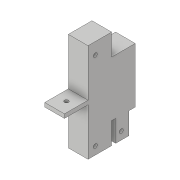
# Autodesk Inventor part: 00_Microlinearmotor
Saved by Autodesk Inventor 2019.4 (Build 234330000, 330)
## iProperties
Created: 2021-09-28
Part Number: 00_Microlinearmotor
Material: Generic
Document SubType Name: Modeling
Designer: diederichbenedict
Density: 1 g/cm^3
Appearance: Default
Author: diederichbenedict
Autodesk Inventor part; units mm, degrees
ref_plane "YZ Plane" through (0, 0, 0) normal (1, 0, 0) x (0, 1, 0)
ref_plane "XZ Plane" through (0, 0, 0) normal (0, 1, 0) x (-1, 0, 0)
ref_plane "XY Plane" through (0, 0, 0) normal (0, 0, 1) x (1, 0, 0)
sketch "Sketch1" plane through (0, 0, 0) normal (1, 0, 0) x (0, 1, 0)
  line L0 (-3.0178, 2.5025) -> (21.9822, 2.5025)
  line L1 (21.9822, 2.5025) -> (21.9822, -3.4975)
  line L2 (21.9822, -3.4975) -> (-3.0178, -3.4975)
  line L3 (-3.0178, -3.4975) -> (-3.0178, 2.5025)
  circle A0 centre (-1.0178, 0.668) radius 0.5
  circle A1 centre (18.9822, 0.668) radius 0.5
  line L4 (16.4822, -3.4975) -> (2.4822, -3.4975)
  line L5 (2.4822, -3.4975) -> (2.4822, -9.4975)
  line L6 (2.4822, -9.4975) -> (16.4822, -9.4975)
  line L7 (9.9822, 2.5025) -> (8.9822, 2.5025)
  line L8 (8.9822, 2.5025) -> (8.9822, 8.5025)
  line L9 (8.9822, 8.5025) -> (9.9822, 8.5025)
  line L10 (9.9822, 8.5025) -> (9.9822, 2.5025)
  line L11 (16.4822, -9.4975) -> (16.4822, -3.4975)
  circle A2 centre (-1.0178, -5.932) radius 0.5
  line L12 (2.4822, -4.5336) -> (-3.0178, -4.5336)
  line L13 (-3.0178, -4.5336) -> (-3.0178, -7.908)
  line L14 (-3.0178, -7.908) -> (2.4822, -7.908)
  line L15 (2.4822, -7.908) -> (2.4822, -4.5336)
  point P0 (0, 0)
  dimension "d0" = 25
  dimension "d1" = 6
  dimension "d2" = 1
  dimension "d3" = 1
  dimension "d4" = 20
  dimension "d5" = 14
  dimension "d6" = 6
  dimension "d8" = 1
  dimension "d9" = 6
  dimension "d10" = 10
  dimension "d13" = 2
  dimension "d18" = 3
  dimension "d19" = 5.5
  dimension "d20" = 1
  dimension "d21" = 6.6
  constraints: 32 end point, 7 parallel, 4 horizontal, 4 perpendicular, 3 centre point, 3 point on line, 1 vertical
  measures "d0" distance of L1.end L2.end
  measures "d1" distance of L0.end L1.end
  measures "d2" diameter of A0
  measures "d3" diameter of A1
  measures "d4" distance of A0.centre A1.centre
  measures "d5" distance of L6.end L5.end
  measures "d6" distance of L5.end L4.end
  measures "d8" distance of L8.end L9.end
  measures "d9" distance of L7.end L8.end
  measures "d10" distance from line of L8 A0.centre
  measures "d13" distance from line of A0.centre L3
  measures "d18" distance from line of A1.centre L1
  measures "d19" distance between parallel lines of L1 L11
  measures "d20" diameter of A2
  measures "d21" distance of A2.centre A0.centre
extrude "Extrusion1" add sketch "Sketch1" along normal blind 5
sketch "Sketch2" plane through (0, 8.9822, 2.5025) normal (0, -1, 0) x (1, 0, 0)
  line L0 (0, 6) -> (0, 0) projected
  line L1 (0, 0) -> (5, 0) projected
  line L2 (5, 6) -> (5, 0) projected
  line L3 (0, 6) -> (5, 6) projected
  circle A0 centre (2.5, 3) radius 0.5
  point P0 (0, -2.5025)
  dimension "d14" = 1
  constraints: 1 centre point
  measures "d14" diameter of A0
extrude "Extrusion2" cut sketch "Sketch2" against normal blind 5 contours A0
body "Solid1"
